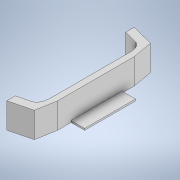
# Autodesk Inventor part: Pala del Robot
Saved by Autodesk Inventor 2022.2 (Build 262287010, 287A)
## iProperties
Created: 2022-03-28
Part Number: Pala del Robot
Material: Generic
Document SubType Name: Modeling
Designer: Santiago Larraín
Density: 1 g/cm^3
Appearance: Default
Author: Santiago Larraín
Autodesk Inventor part; units mm, degrees
ref_plane "YZ Plane" through (0, 0, 0) normal (1, 0, 0) x (0, 1, 0)
ref_plane "XZ Plane" through (0, 0, 0) normal (0, 1, 0) x (-1, 0, 0)
ref_plane "XY Plane" through (0, 0, 0) normal (0, 0, 1) x (1, 0, 0)
sketch "Sketch1" plane through (0, 0, 0) normal (0, 1, 0) x (-1, 0, 0)
  line L0 (15, 80) -> (15, 90)
  line L1 (-15, 0) -> (-15, -30)
  line L2 (-15, 0) -> (-15, 60)
  line L3 (-15, 60) -> (-10.8764, 83.3859)
  line L4 (-15, 60) -> (8.7467, 60) construction
  line L5 (-10.8764, 83.3859) -> (15, 90)
  line L6 (-15, -30) -> (-10.8764, -53.3859)
  line L7 (15, -60) -> (-10.8764, -53.3859)
  line L8 (15, 90) -> (15, 80)
  line L9 (15, 80) -> (0, 76.166)
  line L10 (15, -60) -> (15, -50)
  line L11 (15, -50) -> (-0.3615, -46.0736)
  line L12 (-8, 0) -> (-8, 61.3333)
  line L13 (-8, 0) -> (-8, -31.3333)
  line L14 (0, 76.166) -> (-8, 74.1212) construction
  line L15 (-8, 74.1212) -> (-8, 60) construction
  spline S0 degree 2 poles (0, 76.166) (-8, 74.1212) (-8, 60) knots 1 1 1 2 2 2
  line L16 (-0.3615, -46.0736) -> (-8, -44.1212) construction
  line L17 (-8, -44.1212) -> (-8, -31.3333) construction
  spline S1 degree 2 poles (-0.3615, -46.0736) (-8, -44.1212) (-8, -31.3333) knots 1 1 1 2 2 2
  point P0 (0, 0)
  dimension "d4" = 30
  dimension "d5" = 60
  dimension "d6" = 80
  dimension "d7" = 10
  dimension "d8" = 10
  dimension "d18" = 31.3333
  dimension "d19" = 61.3333
  constraints: 28 end point, 2 collinear, 2 point on line, 1 equal length, 1 horizontal, 1 vertical, 6 other
  measures "d4" distance of L1.start L1.end
  measures "d5" distance of L1.start L2.end
  measures "d6" angle of L4 L3
  measures "d7" distance of L0.start L0.end
  measures "d8" distance of L7.start L10.end
  measures "d18" distance of L12.start L13.end
  measures "d19" distance of L12.start L12.end
extrude "Extrusion1" add sketch "Sketch1" along normal blind 30
sketch "Sketch3" plane through (15, 0, 60) normal (1, 0, 0) x (0, 0, -1)
  line L0 (0, 0) -> (0, 30) projected
  line L1 (0, 0) -> (90, 0) projected
  line L2 (15.6667, 0) -> (75.6667, 0)
  line L3 (75.6667, 0) -> (75.6667, 2)
  line L4 (75.6667, 2) -> (15.6667, 2)
  line L5 (15.6667, 2) -> (15.6667, 0)
  line L6 (91.3333, 0) -> (0, 0) projected
  point P0 (60, 0)
  point P1 (45.6667, 0)
  constraints: 8 end point, 2 point on line, 1 horizontal, 1 midpoint, 1 parallel
extrude "Extrusion3" add sketch "Sketch3" along normal blind 16
body "Solid1"
